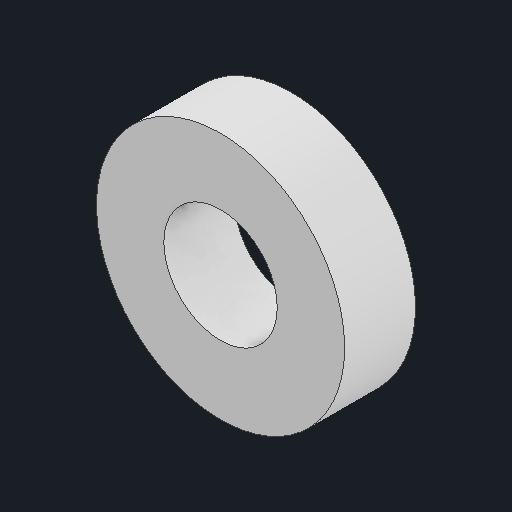
# Autodesk Inventor part: case_top_standoff
Saved by Autodesk Inventor 2022 (Build 260153000, 153)
## iProperties
Created: 2022-04-10
Part Number: case_top_standoff
Material: Generic
Document SubType Name: Modeling
Designer: dvorakj
Density: 1 g/cm^3
Appearance: Default
Author: dvorakj
Autodesk Inventor part; units mm, degrees
ref_plane "YZ Plane" through (0, 0, 0) normal (1, 0, 0) x (0, 1, 0)
ref_plane "XZ Plane" through (0, 0, 0) normal (0, 1, 0) x (-1, 0, 0)
ref_plane "Work Plane1" through (0, 0, 0) normal (0, 0, 1) x (1, 0, 0)
sketch "Sketch1" plane through (0, 0, 0) normal (0, 0, 1) x (1, 0, 0)
  circle A0 centre (-10.8704, 50.5704) radius 3.5
  circle A1 centre (-10.8704, 50.606) radius 1.6
  dimension "d0" = 7
  dimension "d1" = 3.2
  constraints: 2 centre point
  measures "d0" diameter of A0
  measures "d1" diameter of A1
extrude "Extrusion1" add sketch "Sketch1" along normal blind 2
body "Solid1"
